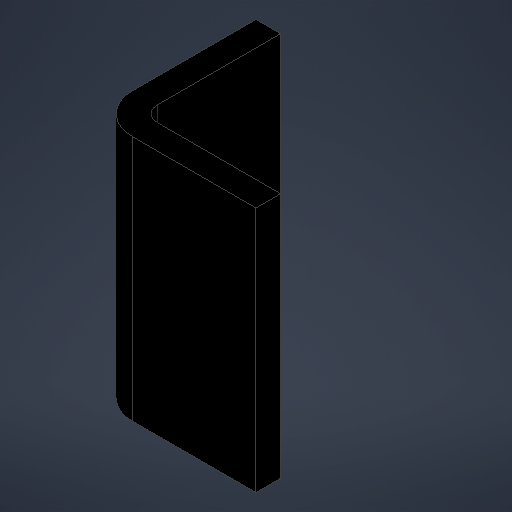
# Autodesk Inventor part: Cylinder holding bracket
Saved by Autodesk Inventor 2027 (Build 310192000, 192)
## iProperties
Created: 2026-04-25
Part Number: Cylinder holding bracket
Material: Generic
Document SubType Name: Modeling
Designer: ratik
Density: 1 g/cm^3
Appearance: Default
Author: ratik
Autodesk Inventor part; units mm, degrees
ref_plane "YZ Plane" through (0, 0, 0) normal (1, 0, 0) x (0, 1, 0)
ref_plane "XZ Plane" through (0, 0, 0) normal (0, 1, 0) x (-1, 0, 0)
ref_plane "XY Plane" through (0, 0, 0) normal (0, 0, 1) x (1, 0, 0)
sketch "Sketch1" plane through (0, 0, 0) normal (0, 1, 0) x (-1, 0, 0)
  line L0 (-3.1194, 0.753) -> (-23.1194, 0.753)
  line L1 (-23.1194, 0.753) -> (-23.1194, -3.247)
  line L2 (-23.1194, -3.247) -> (-3.1194, -3.247)
  line L3 (-0.6194, -5.747) -> (-0.6194, -25.747)
  line L4 (-0.6194, -25.747) -> (3.3806, -25.747)
  line L5 (3.3806, -25.747) -> (3.3806, -5.747)
  arc A0 (-0.6194, -5.747) -> (-3.1194, -3.247) centre (-3.1194, -5.747) ccw
  arc A1 (3.3806, -5.747) -> (-3.1194, 0.753) centre (-3.1194, -5.747) ccw
  point P0 (0, 0)
  dimension "d0" = 20
  dimension "d1" = 4
  dimension "d2" = 4
  dimension "d3" = 20
  dimension "d6" = 2.5
  dimension "d7" = 6.5
  constraints: 12 end point, 4 point on circle, 2 centre point, 2 parallel, 1 horizontal, 1 perpendicular
  measures "d0" distance of L4.end L5.end
  measures "d1" distance of L3.end L4.end
  measures "d2" distance of L0.end L1.end
  measures "d3" distance of L0.start L0.end
  measures "d6" radius of A0
  measures "d7" radius of A1
extrude "Extrusion1" add sketch "Sketch1" along normal blind 40
body "Solid1"
